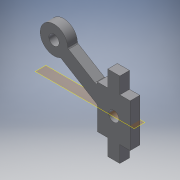
# Autodesk Inventor part: Part18
Saved by Autodesk Inventor 2019.2 (Build 232265000, 265)
## iProperties
Created: 2019-04-03
Part Number: Part18
Material: Generic
Document SubType Name: Modeling
Designer: richard.girt
Mass: 0.649606 g
Surface Area: 7.99472 cm^2
Volume: 0.649606 cm^3
Density: 1 g/cm^3
Appearance: Default
Author: richard.girt
Autodesk Inventor part; units mm, degrees
ref_plane "YZ Plane" through (0, 0, 0) normal (1, 0, 0) x (0, 1, 0)
ref_plane "XZ Plane" through (0, 0, 0) normal (0, 1, 0) x (-1, 0, 0)
ref_plane "XY Plane" through (0, 0, 0) normal (0, 0, 1) x (1, 0, 0)
sketch "Sketch1" plane through (0, 0, 0) normal (0, 0, 1) x (1, 0, 0)
  line L0 (-1.75, 6.25) -> (-4.75, 6.25)
  line L1 (-4.75, 0.2531) -> (-4.75, -6.25)
  line L2 (-4.75, -6.25) -> (-1.75, -6.25)
  line L3 (1.75, -6.25) -> (4.75, -6.25)
  line L4 (4.75, -6.25) -> (4.75, 6.25)
  line L5 (4.75, 6.25) -> (1.75, 6.25)
  line L6 (1.75, -6.25) -> (1.75, -11)
  line L7 (1.75, -11) -> (-1.75, -11)
  line L8 (-1.75, -11) -> (-1.75, -6.25)
  line L9 (-1.75, 6.25) -> (-1.75, 11)
  line L10 (-1.75, 11) -> (1.75, 11)
  line L11 (1.75, 11) -> (1.75, 6.25)
  arc A0 (-13.3683, 10.6806) -> (-15.6681, 6.8774) centre (-17.3643, 10.5) ccw
  circle A1 centre (-17.3643, 10.5) radius 1.5
  circle A2 centre (0, 0) radius 1.5
  line L12 (-17.3643, 10.5) -> (0, 0) construction
  line L13 (-15.1973, 6.8525) -> (-4.9913, 0.681)
  line L14 (-13.1276, 10.2753) -> (-5.5087, 5.6683)
  line L15 (-7.6472, 6.9614) -> (-9.717, 3.5386) construction
  arc A3 (-13.3683, 10.6806) -> (-13.1276, 10.2753) centre (-12.8689, 10.7032) ccw
  arc A4 (-15.1973, 6.8525) -> (-15.6681, 6.8774) centre (-15.4561, 6.4246) ccw
  arc A5 (-4.75, 0.2531) -> (-4.9913, 0.681) centre (-5.25, 0.2531) ccw
  line L16 (-4.75, 6.25) -> (-4.75, 6.0961)
  arc A6 (-5.5087, 5.6683) -> (-4.75, 6.0961) centre (-5.25, 6.0961) ccw
  point P0 (0, 0)
  point P1 (0, 11)
  point P2 (0, -11)
  point P3 (1.75, 8.625)
  point P4 (-15.4349, 6.9961)
  point P5 (-13.3651, 10.419)
  point P6 (-4.75, 5.2095)
  point P7 (-8.6821, 5.25)
  dimension "d0" = 3
  dimension "d1" = 12.5
  dimension "d2" = 9.5
  dimension "d3" = 3.5
  dimension "d4" = 22
  dimension "d5" = 11
  dimension "d6" = 17.3643
  dimension "d7" = 10.5
  dimension "d8" = 3
  dimension "d9" = 8
  dimension "d10" = 4
  dimension "d11" = 0.5
  constraints: 34 end point, 12 point on circle, 8 tangent, 7 centre point, 7 point on line, 6 equal length, 5 midpoint, 5 perpendicular, 4 vertical, 3 equal radius, 3 vertical alignment, 2 parallel, 1 coincident, 1 horizontal
  measures "d0" diameter of A2
  measures "d1" distance of L3.end L4.end
  measures "d2" distance between parallel lines of L1 L4
  measures "d3" distance of L9.end L10.end
  measures "d4" distance between parallel lines of L7 L10
  measures "d5" distance from line of L10 L12.end
  measures "d6" horizontal distance of L12.start L12.end
  measures "d7" vertical distance of L12.start point (0, 0)
  measures "d8" diameter of A1
  measures "d9" diameter of A0
  measures "d10" distance between parallel lines of L13 L14
  measures "d11" radius of A3
extrude "Extrusion1" add sketch "Sketch1" along normal mid plane 2.8
equation "\"d5\" = 0.5 * d4"
body "Solid1"
